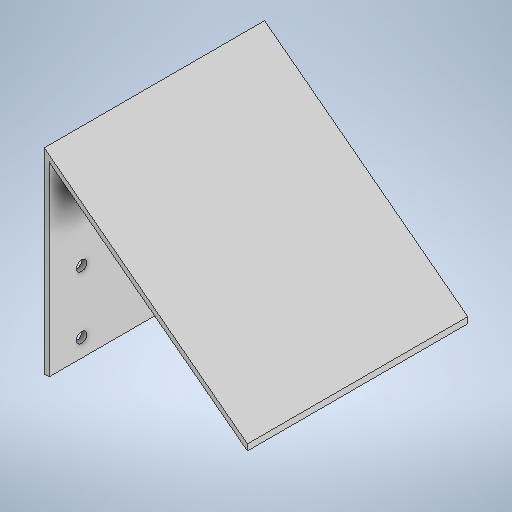
# Autodesk Inventor part: P1D1_2Ramp
Saved by Autodesk Inventor 2025.1 (Build 291241000, 241)
## iProperties
Created: 2024-10-22
Part Number: P1D1_2Ramp
Material: Generic
Document SubType Name: Modeling
Designer: hanna
Density: 1 g/cm^3
Appearance: Default
Author: hanna
Autodesk Inventor part; units mm, degrees
ref_plane "YZ Plane" through (0, 0, 0) normal (1, 0, 0) x (0, 1, 0)
ref_plane "XZ Plane" through (0, 0, 0) normal (0, 1, 0) x (-1, 0, 0)
ref_plane "XY Plane" through (0, 0, 0) normal (0, 0, 1) x (1, 0, 0)
sketch "Sketch1" plane through (0, 0, 0) normal (0, 0, 1) x (1, 0, 0)
  line L0 (0, 0) -> (0, 80)
  line L1 (0, 0) -> (83, 0)
  line L2 (83, 16.7925) -> (83, 0)
  line L3 (0, 80) -> (83, 16.7925)
  dimension "d0" = 80
  dimension "d1" = 83
  constraints: 8 end point, 2 vertical, 1 horizontal
  measures "d0" distance of L0.start L0.end
  measures "d1" distance of L0.start L1.end
extrude "Extrusion1" add sketch "Sketch1" along normal blind 90
shell "Shell1" thickness 2 removed faces 2 at (27.6667, 0, 60) at (83, 5.5975, 30)
sketch "Sketch2" plane through (0, 0, 0) normal (-1, 0, 0) x (0, 0, 1)
  circle A0 centre (13.25, 32.7) radius 2.125
  circle A1 centre (13.25, 7.3) radius 2.125
  circle A2 centre (76.75, 32.7) radius 2.125
  line L0 (90, 80) -> (90, 0) projected
  line L1 (0, 80) -> (0, 0) projected
  circle A3 centre (76.75, 7.3) radius 2.125
  line L2 (0, 0) -> (90, 0) projected
  line L3 (0, 80) -> (90, 80) projected
  circle A4 centre (13.25, 58.1) radius 2.125
  circle A5 centre (76.75, 58.1) radius 2.125
  dimension "d5" = 4.25
  dimension "d6" = 4.25
  dimension "d7" = 4.25
  dimension "d8" = 63.5
  dimension "d10" = 13.25
  dimension "d11" = 25.4
  dimension "d12" = 4.25
  dimension "d13" = 63.5
  dimension "d14" = 7.3
  dimension "d15" = 7.3
  dimension "d28" = 13.25
  dimension "d36" = 4.25
  dimension "d37" = 4.25
  dimension "d38" = 25.4
  dimension "d39" = 25.4
  dimension "d40" = 21.9
  dimension "d41" = 21.9
  dimension "d42" = 13.25
  constraints: 6 centre point
  measures "d5" diameter of A0
  measures "d6" diameter of A1
  measures "d7" diameter of A2
  measures "d8" distance of A2.centre A0.centre
  measures "d10" distance from line of A1.centre L1
  measures "d11" distance of A1.centre A0.centre
  measures "d12" diameter of A3
  measures "d13" distance of A3.centre A1.centre
  measures "d14" distance from line of L2 A1.centre
  measures "d15" distance from line of L2 A3.centre
  measures "d28" distance from line of L0 A2.centre
  measures "d36" diameter of A4
  measures "d37" diameter of A5
  measures "d38" distance of A4.centre A0.centre
  measures "d39" distance of A2.centre A5.centre
  measures "d40" distance from line of L3 A4.centre
  measures "d41" distance from line of L3 A5.centre
  measures "d42" distance from line of L1 A4.centre
extrude "Extrusion2" cut sketch "Sketch2" against normal blind 2 contours A0 | A1 | A2 | A3 | A4 | A5
sketch "Sketch3" plane through (0, 0, 90) normal (0, 0, 1) x (1, 0, 0)
  circle A0 centre (78.5, 8.5093) radius 2.5
  line L0 (83, 0) -> (83, 16.7925) projected
  line L1 (83, 16.7925) -> (0, 80) projected
  point P0 (0, 0)
  point P1 (83, 8.3963)
  dimension "d19" = 5
  dimension "d20" = 4.5
  dimension "d21" = 9.3163
  constraints: 1 centre point, 1 midpoint
  measures "d19" diameter of A0
  measures "d20" horizontal distance of point (83, 8.396) A0.centre
  measures "d21" distance from line of L1 A0.centre
extrude "Extrusion3" cut sketch "Sketch3" against normal blind 2
sketch "Sketch4" plane through (0, 0, 0) normal (0, 0, -1) x (-1, 0, 0)
  circle A0 centre (-78.5, 8.5093) radius 2.5 projected
  circle A1 centre (-78.5, 8.5093) radius 2.5
  point P0 (0, 0)
  dimension "d24" = 5
  constraints: 1 centre point, 1 coincident
  measures "d24" diameter of A1
extrude "Extrusion4" cut sketch "Sketch4" against normal blind 2
sketch "Sketch7" plane through (2, 0, 2) normal (0, 0, 1) x (1, 0, 0)
  line L0 (81, 0) -> (0, 0) projected
  line L1 (0, 75.963) -> (0, 0) projected
  line L2 (0, 0) -> (0, 75.963)
  line L3 (81, 14.2786) -> (81, 0) projected
  line L4 (0, 75.963) -> (81, 14.2786)
  line L5 (81, 14.2786) -> (81, 0)
  line L6 (81, 0) -> (0, 0)
  point P0 (-2, 0)
  constraints: 8 end point, 1 parallel, 1 perpendicular, 1 vertical
extrude "Extrusion7" cut sketch "Sketch7" against normal blind 2
sketch "Sketch8" plane through (83, 0, 88) normal (0, 0, -1) x (-1, 0, 0)
  line L0 (0, 0) -> (0, 14.2786) projected
  line L1 (0, 0) -> (0, 16.7925) projected
  line L2 (0, 14.2786) -> (0, 0)
  line L3 (81, 75.963) -> (81, 0) projected
  line L4 (0, 0) -> (81, 0)
  line L5 (81, 0) -> (81, 75.963)
  line L6 (81, 75.963) -> (0, 14.2786)
  line L7 (0, 16.7925) -> (83, 80) projected
  point P0 (83, 0)
  constraints: 8 end point, 2 perpendicular, 1 parallel, 1 vertical
extrude "Extrusion8" cut sketch "Sketch8" against normal blind 2
body "Solid1"
